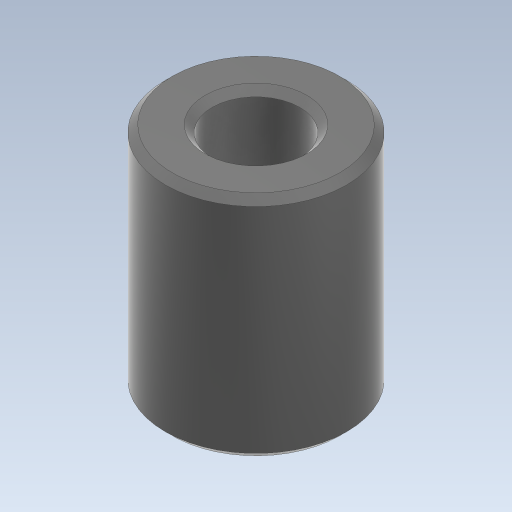
# Autodesk Inventor part: 1lb CF Spring Hub V1
Saved by Autodesk Inventor 2023 (Build 270158000, 158)
## iProperties
Created: 2022-07-22
Part Number: 1lb CF Spring Hub V1
Material: Thermoplastic Resin
Document SubType Name: Modeling
Designer: david
Density: 1.28 g/cm^3
Appearance: Smooth - Black
Author: david
## iProperties of the stored document 1lb CF Spring Hub V1_3DPrint.ipt
Created: 2022-11-09
Part Number: 1lb CF Spring Hub V1_3DPrint
Material: Generic
Document SubType Name: Modeling
Designer: Dave
Density: 1 g/cm^3
Appearance: Default
Author: Dave
Autodesk Inventor part; units mm, degrees
ref_plane "YZ Plane" through (0, 0, 0) normal (1, 0, 0) x (0, 1, 0)
ref_plane "XZ Plane" through (0, 0, 0) normal (0, 1, 0) x (-1, 0, 0)
ref_plane "XY Plane" through (0, 0, 0) normal (0, 0, 1) x (1, 0, 0)
sketch "Sketch1" plane through (0, 0, 0) normal (0, 1, 0) x (-1, 0, 0)
  circle A0 centre (0, 0) radius 2.5
  circle A1 centre (0, 0) radius 5.175
  dimension "d0" = 5
  dimension "d1" = 10.35
  constraints: 2 centre point, 2 coincident
  measures "d0" diameter of A0
  measures "d1" diameter of A1
extrude "Extrusion1" add sketch "Sketch1" along normal blind 13
chamfer "Chamfer1" distance 0.4 angle 45 4 edges at (2.5, 13, 0) (5.175, 13, 0) (5.175, 0, 0) (2.5, 0, 0)
body "Solid1"
